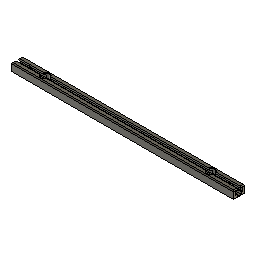
Mounting Bar v8 (Autodesk Fusion 360 design; units mm, degrees)
Autodesk Fusion 360 part; units mm, degrees
note: some values were not read from the file. Set by a fixed rule: which sketch regions a step uses.
sketch "Sketch1" plane through (0, 0, 0) normal (0, 0, 1) x (1, 0, 0)
  line L0 (0, 0) -> (195, 0)
  line L1 (195, 0) -> (195, 10)
  line L2 (195, 10) -> (0, 10)
  line L3 (0, 10) -> (0, 0)
  dimension "d1" = 195
  dimension "d2" = 10
  constraint horizontal L0
  constraint vertical L1
  constraint horizontal L2
  constraint vertical L3
  constraint coincident L0.start L3.end
  measures "d1" distance of L0.start L0.end
  measures "d2" distance of L0.start L2.end
extrude "Extrude1" add sketch "Sketch1" along normal blind 7
sketch "Sketch2" plane through (195, 0, 0) normal (1, 0, 0) x (0, 1, 0)
  line L0 (0, 0) -> (10, 0)
  line L1 (10, 0) -> (10, 7)
  line L2 (10, 7) -> (0, 7)
  line L3 (0, 7) -> (0, 0)
  line L4 (2.1, 5.5) -> (7.9, 5.5)
  line L5 (7.9, 5.5) -> (7.9, 2.9)
  line L6 (7.9, 2.9) -> (2.1, 2.9)
  line L7 (2.1, 2.9) -> (2.1, 5.5)
  line L8 (5, 7) -> (5, 0) construction
  line L9 (5, 5.5) -> (5, 2.9) construction
  line L10 (3.25, 2.9) -> (6.75, 2.9)
  line L11 (6.75, 2.9) -> (6.75, 1.1)
  line L12 (6.75, 1.1) -> (3.25, 1.1)
  line L13 (3.25, 1.1) -> (3.25, 2.9)
  line L14 (3.4, 7) -> (6.6, 7)
  line L15 (6.6, 7) -> (6.6, 5.5)
  line L16 (6.6, 5.5) -> (3.4, 5.5)
  line L17 (3.4, 5.5) -> (3.4, 7)
  dimension "d5" = 5.8
  dimension "d6" = 1.5
  dimension "d7" = 2.6
  dimension "d8" = 3.5
  dimension "d9" = 1.1
  dimension "d10" = 3.2
  constraint horizontal L4
  constraint vertical L5
  constraint horizontal L6
  constraint vertical L7
  constraint midpoint L2 L8.start
  constraint midpoint L0 L8.end
  constraint midpoint L4 L9.start
  constraint midpoint L6 L9.end
  constraint collinear L8 L9
  constraint horizontal L10
  constraint vertical L11
  constraint horizontal L12
  constraint vertical L13
  constraint coincident L6 L10.start
  constraint symmetric L8 L11 L13
  constraint horizontal L14
  constraint vertical L15
  constraint horizontal L16
  constraint vertical L17
  constraint coincident L2 L14.start
  constraint symmetric L8 L15 L17
  constraint collinear L4 L16
  measures "d5" distance of L4.start L4.end
  measures "d6" distance of L2 L4
  measures "d7" distance of L4.end L5.end
  measures "d8" distance of L11.end L12.end
  measures "d9" distance of L0 L12
  measures "d10" distance of L14.start L14.end
extrude "Extrude2" cut sketch "Sketch2" against normal up to surface (195 mm away) contours L2 L4 L14 L15 L16 L17 | L4 L5 L6 L7 L10 L16 | L6 L10 L11 L12 L13
chamfer "Chamfer1" distance 0.4 angle 45 2 edges at (97.5, 7.9, 5.5) (97.5, 2.1, 5.5)
sketch "Sketch3" plane through (0, 0, 2.9) normal (0, 0, 1) x (-1, 0, 0)
  line L0 (0, -7.9) -> (0, -6.75)
  line L1 (0, -6.75) -> (-195, -6.75)
  line L2 (-195, -6.75) -> (-195, -7.9)
  line L3 (-195, -7.9) -> (0, -7.9)
  line L4 (0, -3.25) -> (0, -2.1)
  line L5 (0, -2.1) -> (-195, -2.1)
  line L6 (-195, -2.1) -> (-195, -3.25)
  line L7 (-195, -3.25) -> (0, -3.25)
  line L8 (-185.2, -7.9) -> (-186, -7.9)
  line L9 (-186, -7.9) -> (-186, -2)
  line L10 (-186, -2) -> (-185.2, -2)
  line L11 (-185.2, -2) -> (-185.2, -7.9)
  line L12 (-192.5, -7.9) -> (-193.5, -7.9)
  line L13 (-193.5, -7.9) -> (-193.5, -2.1)
  line L14 (-193.5, -2.1) -> (-192.5, -2.1)
  line L15 (-192.5, -2.1) -> (-192.5, -7.9)
  line L16 (-97.5, -7.9) -> (-97.5, -2.1) construction
  line L17 (-9, -7.9) -> (-9, -2)
  line L18 (-9.8, -2) -> (-9.8, -7.9)
  line L19 (-1.5, -7.9) -> (-1.5, -2.1)
  line L20 (-2.5, -2.1) -> (-2.5, -7.9)
  dimension "d13" = 0.8
  dimension "d14" = 9
  dimension "d15" = 1
  dimension "d16" = 6.5
  constraint horizontal L8
  constraint vertical L9
  constraint horizontal L10
  constraint vertical L11
  constraint coincident L3 L8.start
  constraint horizontal L12
  constraint vertical L13
  constraint horizontal L14
  constraint vertical L15
  constraint coincident L5 L13.end
  constraint coincident L3 L12.start
  constraint midpoint L3 L16.start
  constraint midpoint L5 L16.end
  constraint symmetric L8.start L16 L18.end
  constraint symmetric L8.end L16 L17.start
  constraint symmetric L9.end L16 L17.end
  constraint symmetric L10.end L16 L18.start
  constraint symmetric L12.start L16 L20.end
  constraint symmetric L12.end L16 L19.start
  constraint symmetric L13.end L16 L19.end
  constraint symmetric L14.end L16 L20.start
  measures "d13" distance of L8.start L8.end
  measures "d14" distance of L2 L9
  measures "d15" distance of L12.start L12.end
  measures "d16" distance of L9 L15
extrude "Extrude4" add sketch "Sketch3" along normal blind 0.4 contours L1 L3 L19 L20 | L5 L7 L19 L20 | L1 L3 L12 L13 L15 | L5 L7 L13 L14 L15
extrude "Extrude3" add sketch "Sketch3" along normal up to surface (2.6 mm away) contours L1 L3 L17 L18 | L5 L7 L17 L18 | L1 L3 L8 L9 L11 | L5 L9 L10 L11
fillet "Fillet1" radius 0.4 8 edges at (1.5, 7.325, 3.3) (2.5, 7.325, 3.3) (1.5, 2.675, 3.3) (2.5, 2.675, 3.3) (192.5, 2.675, 3.3) (193.5, 2.675, 3.3) (192.5, 7.325, 3.3) (193.5, 7.325, 3.3)
sketch "Sketch4" plane through (0, 0, 2.9) normal (0, 0, 1) x (-1, 0, 0)
  line L0 (-192.5, -3.25) -> (-9.8, -3.25)
  line L1 (-9.8, -3.25) -> (-9.8, -2.1)
  line L2 (-9.8, -2.1) -> (-192.5, -2.1)
  circle A0 centre (-170, -5) radius 3.25
  line L3 (-195, -10) -> (0, -10) construction
  line L4 (0, 0) -> (-195, 0) construction
  line L5 (-97.5, -10) -> (-97.5, 0) construction
  line L6 (-195, 0) -> (-195, -10) construction
  line L7 (-97.5, -5) -> (-195, -5) construction
  circle A1 centre (-25, -5) radius 3.25
  line L8 (0, -3.25) -> (0, -2.1)
  line L9 (-9, -2.1) -> (-9, -3.25)
  line L10 (-9, -3.25) -> (-2.5, -3.25)
  line L11 (-2.5, -2.1) -> (-9, -2.1)
  line L12 (-2.5, -3.25) -> (-2.5, -2.1)
  line L13 (-192.5, -2.1) -> (-192.5, -3.25)
  line L14 (-1.5, -2.1) -> (-1.5, -3.25)
  line L15 (-1.5, -3.25) -> (0, -3.25)
  line L16 (0, -2.1) -> (-1.5, -2.1)
  dimension "d24" = 6.5
  dimension "d25" = 25
  constraint midpoint L3 L5.start
  constraint midpoint L4 L5.end
  constraint midpoint L5 L7.start
  constraint midpoint L6 L7.end
  constraint coincident A0.centre L7
  constraint symmetric A0 L5 A1
  measures "d24" diameter of A0
  measures "d25" distance of A0.centre L6
extrude "Extrude5" cut sketch "Sketch4" along normal up to surface (4.1 mm away) contours L0 L2 A0 | L0 A0 | L2 A0 | L0 L2 A1 | L0 A1 | L2 A1
chamfer "Chamfer2" distance 0.4 angle 45 4 edges at (97.5, 10, 0) (195, 5, 0) (97.5, 0, 0) (0, 5, 0)
chamfer "Chamfer3" distance 0.8 angle 45 6 edges at (97.5, 0, 7) (97.5, 10, 7) (0, 8.3, 7) (0, 1.7, 7) (195, 8.3, 7) (195, 1.7, 7)
chamfer "Chamfer4" distance 0.3 angle 45 20 edges at (0, 7.325, 2.9) (0, 7.9, 4) (0, 7.7, 5.3) (0, 7.05, 5.5) (0, 2.95, 5.5) (0, 2.3, 5.3) (0, 2.1, 4) (0, 2.675, 2.9) (25, 8.25, 7) (25, 1.75, 7) (170, 1.75, 7) (170, 8.25, 7) (195, 2.675, 2.9) (195, 2.1, 4) (195, 2.3, 5.3) (195, 2.95, 5.5) (195, 7.05, 5.5) (195, 7.7, 5.3) (195, 7.9, 4) (195, 7.325, 2.9)
ref_plane "WorkPlane1" through (35.5, 5, 3.5) normal (-1, 0, 0) x (0, -1, 0)
split "Split1" [suppressed]
